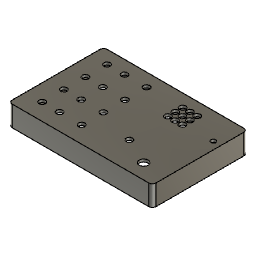
MVP-Version_DesignX2 v3 (Autodesk Fusion 360 design; units mm, degrees)
Autodesk Fusion 360 part; units mm, degrees
sketch "Skizze1" plane through (0, 0, 0) normal (0, 0, 1) x (1, 0, 0)
  line L0 (0, 0) -> (153.266, 0)
  line L1 (153.266, 0) -> (153.266, 98.489)
  line L2 (153.266, 98.489) -> (0, 98.489)
  line L3 (0, 98.489) -> (0, 0)
  line L4 (0, 98.489) -> (7.779, 98.489)
  circle A0 centre (7.779, 92.6815) radius 2.25
  circle A1 centre (76.633, 92.6815) radius 2.25
  circle A2 centre (145.487, 92.6815) radius 2.25
  circle A3 centre (7.779, 49.2445) radius 2.25
  circle A4 centre (7.779, 5.8075) radius 2.25
  circle A5 centre (76.633, 49.2445) radius 2.25
  circle A6 centre (145.487, 49.2445) radius 2.25
  circle A7 centre (76.633, 5.8075) radius 2.25
  circle A8 centre (145.487, 5.8075) radius 2.25
  circle A9 centre (14.7, 87.686) radius 3.5
  circle A10 centre (14.7, 63.406) radius 3.5
  circle A11 centre (14.7, 39.126) radius 3.5
  circle A12 centre (14.7, 14.847) radius 3.5
  circle A13 centre (34.29, 87.686) radius 3.5
  circle A14 centre (34.29, 63.406) radius 3.5
  circle A15 centre (34.29, 39.126) radius 3.5
  circle A16 centre (34.29, 14.847) radius 3.5
  circle A17 centre (59.055, 87.686) radius 3.5
  circle A18 centre (59.055, 63.406) radius 3.5
  circle A19 centre (59.055, 39.126) radius 3.5
  circle A20 centre (59.055, 14.847) radius 3.5
  circle A21 centre (100.4, 26.9865) radius 3.5
  circle A22 centre (130.566, 12.9) radius 5
  circle A23 centre (148.866, 72.939) radius 2.7
  circle A24 centre (115.336, 88.139) radius 3.5
  circle A25 centre (115.336, 79.839) radius 3.5
  circle A26 centre (115.336, 71.539) radius 3.5
  circle A27 centre (107.236, 88.139) radius 3.5
  circle A28 centre (107.236, 79.839) radius 3.5
  circle A29 centre (107.236, 71.539) radius 3.5
  circle A30 centre (99.136, 88.139) radius 3.5
  circle A31 centre (99.136, 79.839) radius 3.5
  circle A32 centre (99.136, 71.539) radius 3.5
  line L5 (-1, 99.489) -> (154.266, 99.489)
  line L6 (154.266, 99.489) -> (154.266, -1)
  line L7 (154.266, -1) -> (-1, -1)
  line L8 (-1, -1) -> (-1, 99.489)
  line L9 (0, 102.489) -> (153.266, 102.489)
  line L10 (157.266, 98.489) -> (157.266, 0)
  line L11 (153.266, -4) -> (0, -4)
  line L12 (-4, 0) -> (-4, 98.489)
  arc A33 (153.266, -4) -> (157.266, 0) centre (153.266, 0) ccw
  arc A34 (157.266, 98.489) -> (153.266, 102.489) centre (153.266, 98.489) ccw
  arc A35 (0, 102.489) -> (-4, 98.489) centre (0, 98.489) ccw
  arc A36 (-4, 0) -> (0, -4) centre (0, 0) ccw
  dimension "d1" = 153.266
  dimension "d2" = 98.489
  dimension "d5" = 7.779
  dimension "d7" = 4.5
  dimension "d8" = 4.5
  dimension "d9" = 4.5
  dimension "d10" = 4.5
  dimension "d11" = 4.5
  dimension "d12" = 4.5
  dimension "d13" = 4.5
  dimension "d14" = 4.5
  dimension "d15" = 4.5
  dimension "d23" = 7
  dimension "d24" = 7
  dimension "d25" = 7
  dimension "d26" = 7
  dimension "d27" = 7
  dimension "d28" = 7
  dimension "d29" = 7
  dimension "d30" = 7
  dimension "d31" = 7
  dimension "d32" = 7
  dimension "d33" = 7
  dimension "d34" = 7
  dimension "d37" = 7
  dimension "d40" = 10
  dimension "d43" = 5.4
  dimension "d46" = 7
  dimension "d47" = 7
  dimension "d48" = 7
  dimension "d49" = 7
  dimension "d50" = 7
  dimension "d51" = 7
  dimension "d52" = 7
  dimension "d53" = 7
  dimension "d54" = 7
  dimension "d67" = 4
  dimension "d68" = 4
  dimension "d69" = 4
  dimension "d70" = 4
  constraint horizontal L0
  constraint vertical L1
  constraint horizontal L2
  constraint vertical L3
  constraint coincident L0.start L3.end
  constraint horizontal L5
  constraint vertical L6
  constraint horizontal L7
  constraint vertical L8
  constraint horizontal L9
  constraint vertical L10
  constraint horizontal L11
  constraint vertical L12
  constraint tangent L11 A33
  constraint tangent L10 A33
  constraint tangent L9 A34
  constraint tangent L10 A34
  constraint tangent L9 A35
  constraint tangent L12 A35
  constraint tangent L12 A36
  constraint tangent L11 A36
  measures "d1" distance of L0.start L0.end
  measures "d2" distance of L0.start L2.end
  measures "d5" distance of L2.end L4.end
  measures "d7" diameter of A0
  measures "d8" diameter of A1
  measures "d9" diameter of A2
  measures "d10" diameter of A3
  measures "d11" diameter of A4
  measures "d12" diameter of A5
  measures "d13" diameter of A6
  measures "d14" diameter of A7
  measures "d15" diameter of A8
  measures "d23" diameter of A9
  measures "d24" diameter of A10
  measures "d25" diameter of A11
  measures "d26" diameter of A12
  measures "d27" diameter of A13
  measures "d28" diameter of A14
  measures "d29" diameter of A15
  measures "d30" diameter of A16
  measures "d31" diameter of A17
  measures "d32" diameter of A18
  measures "d33" diameter of A19
  measures "d34" diameter of A20
  measures "d37" diameter of A21
  measures "d40" diameter of A22
  measures "d43" diameter of A23
  measures "d46" diameter of A24
  measures "d47" diameter of A25
  measures "d48" diameter of A26
  measures "d49" diameter of A27
  measures "d50" diameter of A28
  measures "d51" diameter of A29
  measures "d52" diameter of A30
  measures "d53" diameter of A31
  measures "d54" diameter of A32
  measures "d67" radius of A33
  measures "d68" radius of A34
  measures "d69" radius of A35
  measures "d70" radius of A36
extrude "Extrusion2" add sketch "Skizze1" along normal blind 3 contours L0 L1 L2 L3 L4 | A0 | A1 | A2 | A3 | A4 | A5 | A6 | A7 | A8 | L5 L6 L7 L8 | L9 L10 L11 L12 A33 A34 A35 A36
extrude "Extrusion3" add sketch "Skizze1" against normal blind 20 contours L9 L10 L11 L12 A33 A34 A35 A36
